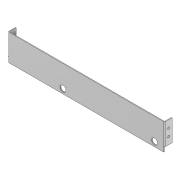
# Autodesk Inventor part: Pared de Refrigeración
Saved by Autodesk Inventor 2020 (Build 240168000, 168)
## iProperties
Created: 2020-09-27
Part Number: Pared de Refrigeración
Material: Aluminum 1100-H14
Document SubType Name: Modeling
Designer: Dante
Density: 2.7 g/cm^3
Appearance: Satin
Author: Dante
Autodesk Inventor part; units mm, degrees
ref_plane "YZ Plane" through (0, 0, 0) normal (1, 0, 0) x (0, 1, 0)
ref_plane "XZ Plane" through (0, 0, 0) normal (0, 1, 0) x (-1, 0, 0)
ref_plane "XY Plane" through (0, 0, 0) normal (0, 0, 1) x (1, 0, 0)
sketch "Sketch1" plane through (0, 0, 0) normal (0, 0, 1) x (1, 0, 0)
  line L0 (0, -18) -> (0, -78)
  line L1 (0, -78) -> (19, -78)
  line L2 (19, -78) -> (19, -18)
  line L3 (19, -18) -> (0, -18)
  line L4 (19, -18) -> (447, -18)
  line L5 (447, -18) -> (447, -78)
  line L6 (447, -78) -> (19, -78)
  line L7 (447, -18) -> (466, -18)
  line L8 (466, -18) -> (466, -78)
  line L9 (466, -78) -> (447, -78)
  circle A0 centre (10, -58) radius 3
  circle A1 centre (10, -38) radius 3
  circle A2 centre (456, -58) radius 3
  circle A3 centre (456, -38) radius 3
  line L10 (19, -78) -> (19, -91)
  line L11 (19, -91) -> (447, -91)
  line L12 (447, -91) -> (447, -78)
  circle A4 centre (169, -78) radius 8
  circle A5 centre (422, -78) radius 8
  dimension "d0" = 60
  dimension "d1" = 19
  dimension "d2" = 428
  dimension "d3" = 19
  dimension "d10" = 6
  dimension "d11" = 6
  dimension "d12" = 20
  dimension "d13" = 20
  dimension "d14" = 6
  dimension "d15" = 6
  dimension "d16" = 20
  dimension "d17" = 20
  dimension "d24" = 13
  dimension "d25" = 428
  dimension "d27" = 10
  dimension "d28" = 10
  dimension "d29" = 10
  dimension "d30" = 10
  dimension "d32" = 16
  dimension "d33" = 13
  dimension "d34" = 150
  dimension "d35" = 16
  dimension "d36" = 25
  constraints: 26 end point, 8 perpendicular, 6 centre point, 2 horizontal, 2 vertical, 1 point on line
  measures "d0" distance of L0.start L0.end
  measures "d1" distance of L0.end L1.end
  measures "d2" distance of L2.end L4.end
  measures "d3" distance of L4.end L7.end
  measures "d10" diameter of A0
  measures "d11" diameter of A1
  measures "d12" distance from line of L1 A0.centre
  measures "d13" distance from line of A1.centre L3
  measures "d14" diameter of A2
  measures "d15" diameter of A3
  measures "d16" distance from line of A2.centre L9
  measures "d17" distance from line of A3.centre L7
  measures "d24" distance of L1.end L10.end
  measures "d25" distance of L10.end L11.end
  measures "d27" distance from line of L0 A1.centre
  measures "d28" distance from line of L0 A0.centre
  measures "d29" distance from line of A3.centre L8
  measures "d30" distance from line of A2.centre L8
  measures "d32" diameter of A4
  measures "d33" distance from line of A4.centre L11
  measures "d34" distance from line of A4.centre L2
  measures "d35" diameter of A5
  measures "d36" distance from line of L5 A5.centre
extrude "Extrusion1" add sketch "Sketch1" along normal blind 2 contours L3 L2 L1 L0
extrude "Extrusion2" add sketch "Sketch1" along normal blind 2 contours L4 L5 L6 A5 A4 L2 | L6 A4 A5 L12 L11 L10
extrude "Extrusion3" add sketch "Sketch1" along normal blind 2 contours L7 L8 L9 L5
bend part "Bend Part2" radius 0.5 angle 90 line through (447, -18, 0) along (0, -1, 0) centre toward (0, 0, -1) moving side (1, 0, 0) both sides no
bend part "Bend Part3" radius 0.5 angle 90 line through (19, -78, 0) along (0, 1, 0) centre toward (0, 0, -1) moving side (-1, 0, 0) both sides no
equation "\"d1\" = d3"
equation "\"d12\" = d13"
equation "\"d16\" = d13"
equation "\"d17\" = d13"
equation "\"d25\" = d2"
equation "\"d28\" = d27"
equation "\"d29\" = d27"
body "Solid1"
